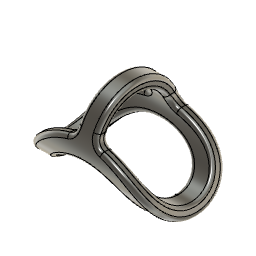
Presidio_dito_ver_1.1 (Autodesk Fusion 360 design; units mm, degrees)
Autodesk Fusion 360 part; units mm, degrees
sketch "Schizzo1" plane through (0, 0, 0) normal (1, 0, 0) x (0, 1, 0)
  circle A0 centre (0, 0) radius 8.5
  circle A1 centre (0, 0) radius 11.5
  dimension "d1" = 3
  dimension "d5" = 17
  constraint coincident A0.centre A1.centre
  measures "d1" distance of A0 A1
  measures "d5" diameter of A0
extrude "Estrusione1" add sketch "Schizzo1" along normal mid plane 36
sketch "Schizzo2" plane through (0, 0, 0) normal (0, 1, 0) x (1, 0, 0)
  line L0 (-18, 11.5) -> (-18, -11.5)
  line L1 (18, -11.5) -> (18, 11.5)
  line L2 (0, 0) -> (0, 28.416826) construction
  circle A0 centre (0, 16.005795) radius 18.555382
  line L3 (0, -11.5) -> (0, 11.5)
  circle A1 centre (0, 16.005795) radius 13.555382
  line L4 (-18, -11.5) -> (0, -11.5)
  line L5 (18, -11.5) -> (0, -11.5)
  line L6 (-2.5, -2.380401) -> (-2.5, -11.5)
  line L7 (2.5, -11.5) -> (2.5, -2.380401)
  point P0 (0, -2.549587)
  dimension "d8" = 14.049587
  dimension "d9" = 5
  dimension "d10" = 5
  constraint coincident L2.start origin
  constraint parallel L1 L2
  constraint coincident L1.end A0
  constraint concentric A0 A1
  constraint coincident L0.end L4.start
  constraint coincident L3.start L4.end
  constraint coincident L1.start L5.start
  constraint coincident L4 L6.end
  constraint perpendicular L4 L6
  constraint coincident L5 L7.start
  constraint perpendicular L5 L7
  constraint equal L6 L7
  measures "d9" distance of A0 A1
  measures "d10" distance of L6 L7
extrude "Estrusione2" cut sketch "Schizzo2" along normal mid plane 36 contours L0 A0 L4 L6 | L1 A0 L5 L7 | A1 picked at (-9.427103, -7.946396) picked at (9.427103, -7.946396) picked at (-1.804153, 13.667479)
fillet "Raccordo1" radius 2.5 4 edges at (-2.5, 9.705412, 2.380401) (-2.5, -9.705412, 2.380401) (2.5, 9.705412, 2.380401) (2.5, -9.705412, 2.380401)
fillet "Raccordo2" radius 1 20 edges at (-3.016338, -11.12125, 2.926727) (-15.144767, -10.21153, -5.286219) (-15.144767, 10.21153, -5.286219) (-3.016101, 11.12115, 2.927092) (-2.5, 0, 11.5) (15.144767, -10.21153, -5.286219) (15.144767, 10.21153, -5.286219) (3.016101, 11.12115, 2.927092) (2.5, 0, 11.5) (3.016101, -11.12115, 2.927092) (-2.996659, -7.970379, 2.953003) (-2.5, 0, 8.5) (-2.997117, 7.970657, 2.952285) (-16.969538, 0, -8.5) (12.784607, 0, -11.5) (-11.287666, 0, -8.5) (2.996659, 7.970379, 2.953003) (2.5, 0, 8.5) (2.996659, -7.970379, 2.953003) (16.969538, 0, -8.5)
equation "d1 = spessore_presidio"
equation "spessore_presidio = 3 mm" comment "Modificare questo valore per aumentare o diminuire lo spessore del presidio.(Valore di default 3.00 mm)"
equation "larghezza_dito = 17 mm" comment "Modificare questo valore in base alla larghezza del dito. (Valore di default 17.00 mm)"
equation "lunghezza_presidio = 36 mm" comment "Modificare questo valore per allungare o accorciare il presidio. (Valore di default 36.00 mm)"
equation "d5 = larghezza_dito"
equation "d6 = lunghezza_presidio"
equation "d8 = larghezza_dito / 1.21"
equation "d9 = spessore_longitudinale"
equation "d10 = spessore_longitudinale"
equation "spessore_longitudinale = 5 mm" comment "Modificare questo valore per aumentare o diminuire lo spessore longitudinale del presidio. (Valore di default 5.00 mm)"
equation "d12 = lunghezza_presidio"
equation "d15 = spessore_longitudinale / 2"
equation "d17 = spessore_presidio / 3"
named bodies: "presidio_dito"
